Autodesk Fusion 360 part; units mm, degrees
(part 2 of 2)
sketch "Sketch18" plane through (0, 0, 0) normal (0, 0, -1) x (1, 0, 0)
  line L0 (46, -5.5) -> (46, -9.25)
  line L1 (46, -9.25) -> (49.5, -10.5)
  line L2 (49.5, -10.5) -> (65.5, -10.5)
  line L3 (65.5, -10.5) -> (65.5, 45.5)
  line L4 (65.5, 45.5) -> (40.5, 80.5)
  line L5 (40.5, 80.5) -> (-10.5, 80.5)
  line L6 (-10.5, 80.5) -> (-35.5, 45.5)
  line L7 (-35.5, 45.5) -> (-35.5, -10.5)
  line L8 (-35.5, -10.5) -> (-19.5, -10.5)
  line L9 (-19.5, -10.5) -> (-16, -9.25)
  line L10 (-16, -9.25) -> (-16, -5.5)
  line L11 (-16, -5.5) -> (46, -5.5)
  line L12 (35.5, 12.5) -> (33, 24.5)
  line L13 (33, 24.5) -> (49.5, 29.5)
  line L14 (49.5, 29.5) -> (49.5, 5.5)
  line L15 (49.5, 5.5) -> (35.5, 12.5)
  line L16 (27, 75.5) -> (35.5, 75.5)
  line L17 (35.5, 75.5) -> (35.5, 64.5)
  line L18 (35.5, 64.5) -> (27, 64.5)
  line L19 (27, 64.5) -> (27, 75.5)
  line L20 (54.5, 0.5) -> (60.5, 0.5)
  line L21 (60.5, 0.5) -> (60.5, -5.5)
  line L22 (60.5, -5.5) -> (54.5, -5.5)
  line L23 (54.5, -5.5) -> (54.5, 0.5)
  line L24 (54.5, 40.5) -> (60.5, 40.5)
  line L25 (60.5, 40.5) -> (60.5, 34.5)
  line L26 (60.5, 34.5) -> (54.5, 34.5)
  line L27 (54.5, 34.5) -> (54.5, 40.5)
  line L28 (-30.5, 0.5) -> (-24.5, 0.5)
  line L29 (-24.5, 0.5) -> (-24.5, -5.5)
  line L30 (-24.5, -5.5) -> (-30.5, -5.5)
  line L31 (-30.5, -5.5) -> (-30.5, 0.5)
  line L32 (-0.5, 7.5) -> (7.5, 7.5)
  line L33 (7.5, 7.5) -> (7.5, -0.5)
  line L34 (7.5, -0.5) -> (-0.5, -0.5)
  line L35 (-0.5, -0.5) -> (-0.5, 7.5)
  line L36 (2, 35.5) -> (28, 35.5)
  line L37 (28, 35.5) -> (28, 29.5)
  line L38 (28, 29.5) -> (2, 29.5)
  line L39 (2, 29.5) -> (2, 35.5)
  line L40 (-30.5, 40.5) -> (-24.5, 40.5)
  line L41 (-24.5, 40.5) -> (-24.5, 34.5)
  line L42 (-24.5, 34.5) -> (-30.5, 34.5)
  line L43 (-30.5, 34.5) -> (-30.5, 40.5)
  line L44 (22.5, 7.5) -> (30.5, 7.5)
  line L45 (30.5, 7.5) -> (30.5, -0.5)
  line L46 (30.5, -0.5) -> (22.5, -0.5)
  line L47 (22.5, -0.5) -> (22.5, 7.5)
  line L48 (-5.5, 75.5) -> (3, 75.5)
  line L49 (3, 75.5) -> (3, 64.5)
  line L50 (3, 64.5) -> (-5.5, 64.5)
  line L51 (-5.5, 64.5) -> (-5.5, 75.5)
  line L52 (33, 40.5) -> (-3, 40.5)
  line L53 (-3, 40.5) -> (8, 59.5)
  line L54 (8, 59.5) -> (22, 59.5)
  line L55 (22, 59.5) -> (33, 40.5)
  line L56 (-5.5, 12.5) -> (-19.5, 5.5)
  line L57 (-19.5, 5.5) -> (-19.5, 29.5)
  line L58 (-19.5, 29.5) -> (-3, 24.5)
  line L59 (-3, 24.5) -> (-5.5, 12.5)
  line L60 (30.5, -0.5) -> (35.5, -0.5) construction
  line L61 (35.5, -0.5) -> (35.5, -5.5) construction
  line L62 (35.5, -5.5) -> (30.5, -5.5) construction
  line L63 (30.5, -5.5) -> (30.5, -0.5) construction
  line L64 (35.5, -5.5) -> (17.5, -5.5) construction
  line L65 (17.5, -5.5) -> (17.5, 12.5) construction
  line L66 (17.5, 12.5) -> (35.5, 12.5) construction
  line L67 (35.5, 12.5) -> (35.5, -5.5) construction
  line L68 (7.5, -0.5) -> (12.5, -0.5) construction
  line L69 (12.5, -0.5) -> (12.5, -5.5) construction
  line L70 (12.5, -5.5) -> (7.5, -5.5) construction
  line L71 (7.5, -5.5) -> (7.5, -0.5) construction
  line L72 (12.5, -5.5) -> (-5.5, -5.5) construction
  line L73 (-5.5, -5.5) -> (-5.5, 12.5) construction
  line L74 (-5.5, 12.5) -> (12.5, 12.5) construction
  line L75 (12.5, 12.5) -> (12.5, -5.5) construction
  line L76 (-24.5, -5.5) -> (-19.5, -5.5) construction
  line L77 (-19.5, -5.5) -> (-19.5, -10.5) construction
  line L78 (-19.5, -10.5) -> (-24.5, -10.5) construction
  line L79 (-24.5, -10.5) -> (-24.5, -5.5) construction
  line L80 (-19.5, -10.5) -> (-35.5, -10.5) construction
  line L81 (-35.5, -10.5) -> (-35.5, 5.5) construction
  line L82 (-35.5, 5.5) -> (-19.5, 5.5) construction
  line L83 (-19.5, 5.5) -> (-19.5, -10.5) construction
  line L84 (-19.5, 29.5) -> (-35.5, 29.5)
  line L85 (-35.5, 29.5) -> (-35.5, 5.5)
  line L86 (-35.5, 5.5) -> (-19.5, 5.5)
  line L87 (-19.5, 5.5) -> (-19.5, 29.5)
  line L88 (49.5, 29.5) -> (65.5, 29.5)
  line L89 (65.5, 29.5) -> (65.5, 5.5)
  line L90 (65.5, 5.5) -> (49.5, 5.5)
  line L91 (49.5, 5.5) -> (49.5, 29.5)
  line L92 (60.5, 34.5) -> (65.5, 34.5) construction
  line L93 (65.5, 34.5) -> (65.5, 29.5) construction
  line L94 (65.5, 29.5) -> (60.5, 29.5) construction
  line L95 (60.5, 29.5) -> (60.5, 34.5) construction
  line L96 (65.5, 29.5) -> (49, 29.5) construction
  line L97 (49, 29.5) -> (49, 46) construction
  line L98 (49, 46) -> (65.5, 46) construction
  line L99 (65.5, 46) -> (65.5, 29.5) construction
  line L100 (27, 75.5) -> (22, 75.5) construction
  line L101 (22, 75.5) -> (22, 80.5) construction
  line L102 (22, 80.5) -> (27, 80.5) construction
  line L103 (27, 80.5) -> (27, 75.5) construction
  line L104 (22, 80.5) -> (40.5, 80.5) construction
  line L105 (40.5, 80.5) -> (40.5, 59.5) construction
  line L106 (40.5, 59.5) -> (22, 59.5) construction
  line L107 (22, 59.5) -> (22, 80.5) construction
  line L108 (49, 29.5) -> (31.25, 59.5)
  line L109 (40.5, 80.5) -> (40.5, 59.5)
  line L110 (40.5, 59.5) -> (31.25, 59.5)
  line L111 (-5.5, 75.5) -> (-10.5, 75.5) construction
  line L112 (-10.5, 75.5) -> (-10.5, 80.5) construction
  line L113 (-10.5, 80.5) -> (-5.5, 80.5) construction
  line L114 (-5.5, 80.5) -> (-5.5, 75.5) construction
  line L115 (-10.5, 80.5) -> (8, 80.5) construction
  line L116 (8, 80.5) -> (8, 59.5) construction
  line L117 (8, 59.5) -> (-10.5, 59.5) construction
  line L118 (-10.5, 59.5) -> (-10.5, 80.5) construction
  line L119 (22, 59.5) -> (8, 59.5)
  line L120 (8, 59.5) -> (8, 80.5)
  line L121 (8, 80.5) -> (22, 80.5)
  line L122 (22, 80.5) -> (22, 59.5)
  line L123 (-35.5, 29.5) -> (-19.5, 29.5) construction
  line L124 (-19.5, 29.5) -> (-19.5, 45.5) construction
  line L125 (-19.5, 45.5) -> (-35.5, 45.5) construction
  line L126 (-35.5, 45.5) -> (-35.5, 29.5) construction
  line L127 (-19.5, 29.5) -> (-1.25, 59.5)
  line L128 (49, 29.5) -> (49, 46)
  line L129 (49, 46) -> (65.5, 46)
  line L130 (-1.25, 59.5) -> (-10.5, 59.5)
  line L131 (-10.5, 59.5) -> (-10.5, 80.5)
  line L132 (-19.5, 29.5) -> (-19.5, 45.5)
  line L133 (-19.5, 45.5) -> (-35.5, 45.5)
  line L134 (49, 46) -> (-19.5, 45.5)
  line L135 (49, 46) -> (-19.5, 45.5)
  dimension "d166" = 5
  dimension "d167" = 5
  dimension "d168" = 18
  dimension "d169" = 18
  dimension "d170" = 5
  dimension "d171" = 18
  dimension "d172" = 18
  dimension "d173" = 16
  dimension "d174" = 16
  dimension "d175" = 16.5
  dimension "d176" = 16.5
  dimension "d177" = 5
  dimension "d178" = 18.5
  dimension "d179" = 21
  dimension "d180" = 18.5
  dimension "d181" = 21
  dimension "d182" = 16
  dimension "d183" = 16
  constraint horizontal L60
  constraint vertical L61
  constraint horizontal L62
  constraint vertical L63
  constraint coincident L45.end L46.start
  constraint horizontal L64
  constraint vertical L65
  constraint horizontal L66
  constraint vertical L67
  constraint horizontal L68
  constraint vertical L69
  constraint horizontal L70
  constraint vertical L71
  constraint coincident L33.end L34.start
  constraint horizontal L72
  constraint vertical L73
  constraint horizontal L74
  constraint vertical L75
  constraint horizontal L76
  constraint vertical L77
  constraint horizontal L78
  constraint vertical L79
  constraint coincident L8.end L9.start
  constraint coincident L29.end L30.start
  constraint horizontal L80
  constraint vertical L81
  constraint horizontal L82
  constraint vertical L83
  constraint horizontal L84
  constraint vertical L85
  constraint horizontal L86
  constraint vertical L87
  constraint coincident L57.end L58.start
  constraint horizontal L88
  constraint vertical L89
  constraint horizontal L90
  constraint vertical L91
  constraint coincident L3 L89.end
  constraint coincident L13.end L14.start
  constraint horizontal L92
  constraint vertical L93
  constraint horizontal L94
  constraint vertical L95
  constraint coincident L25.end L26.start
  constraint horizontal L96
  constraint vertical L97
  constraint horizontal L98
  constraint vertical L99
  constraint horizontal L100
  constraint vertical L101
  constraint horizontal L102
  constraint vertical L103
  constraint coincident L16.start L19.end
  constraint horizontal L104
  constraint vertical L105
  constraint horizontal L106
  constraint vertical L107
  constraint midpoint L106 L108.end
  constraint horizontal L111
  constraint vertical L112
  constraint horizontal L113
  constraint vertical L114
  constraint coincident L5.end L6.start
  constraint coincident L48.start L51.end
  constraint horizontal L115
  constraint vertical L116
  constraint horizontal L117
  constraint vertical L118
  constraint horizontal L119
  constraint vertical L120
  constraint horizontal L121
  constraint vertical L122
  constraint coincident L54.end L55.start
  constraint horizontal L123
  constraint vertical L124
  constraint horizontal L125
  constraint vertical L126
  constraint midpoint L117 L127.end
  constraint coincident L6.end L7.start
  measures "d166" distance of L45.end L60.end
  measures "d167" distance of L45.end L62.end
  measures "d168" distance of L61.end L64.end
  measures "d169" distance of L61.end L12.start
  measures "d170" distance of L33.end L68.end
  measures "d171" distance of L69.end L72.end
  measures "d172" distance of L69.end L74.end
  measures "d173" distance of L8.end L7.end
  measures "d174" distance of L8.end L56.end
  measures "d175" distance of L88.end L96.end
  measures "d176" distance of L88.end L98.end
  measures "d177" distance of L16.start L100.end
  measures "d178" distance of L101.end L4.end
  measures "d179" distance of L101.end L54.end
  measures "d180" distance of L5.end L115.end
  measures "d181" distance of L5.end L117.end
  measures "d182" distance of L84.end L57.end
  measures "d183" distance of L84.end L6.end
extrude "Extrude22" cut sketch "Sketch18" against normal blind 6 contours L3 L14 L88 L89 L90 L91 | L7 L57 L84 L85 L86 L87 | L4 L108 L109 L110 L129 L134 L135 | L6 L127 L130 L131 L133 L134 L135 | L5 L54 L119 L120 L121 L122
sketch "Sketch19" plane through (0, 0, 0) normal (0, 0, -1) x (1, 0, 0)
  line L0 (40.5, 59.5) -> (40.5, 80.5)
  line L1 (40.5, 80.5) -> (22, 80.5)
  line L2 (22, 80.5) -> (22, 59.5)
  line L3 (22, 59.5) -> (33, 40.5)
  line L4 (33, 40.5) -> (-3, 40.5)
  line L5 (-3, 40.5) -> (8, 59.5)
  line L6 (8, 59.5) -> (8, 80.5)
  line L7 (8, 80.5) -> (-10.5, 80.5)
  line L8 (-10.5, 80.5) -> (-10.5, 59.5)
  line L9 (-10.5, 59.5) -> (-1.25, 59.5)
  line L10 (-1.25, 59.5) -> (-9.7233, 45.5714)
  line L11 (-9.7233, 45.5714) -> (-19.5, 45.5)
  line L12 (-19.5, 45.5) -> (-35.5, 45.5)
  line L13 (-35.5, 45.5) -> (-35.5, 29.5)
  line L14 (-35.5, 29.5) -> (-19.5, 29.5)
  line L15 (-19.5, 29.5) -> (-3, 24.5)
  line L16 (-3, 24.5) -> (-5.5, 12.5)
  line L17 (-5.5, 12.5) -> (-19.5, 5.5)
  line L18 (-19.5, 5.5) -> (-35.5, 5.5)
  line L19 (-35.5, 5.5) -> (-35.5, -10.5)
  line L20 (-35.5, -10.5) -> (-19.5, -10.5)
  line L21 (-19.5, -10.5) -> (-16, -9.25)
  line L22 (-16, -9.25) -> (-16, -5.5)
  line L23 (-16, -5.5) -> (46, -5.5)
  line L24 (46, -5.5) -> (46, -9.25)
  line L25 (46, -9.25) -> (49.5, -10.5)
  line L26 (49.5, -10.5) -> (65.5, -10.5)
  line L27 (65.5, -10.5) -> (65.5, 5.5)
  line L28 (65.5, 5.5) -> (49.5, 5.5)
  line L29 (49.5, 5.5) -> (35.5, 12.5)
  line L30 (35.5, 12.5) -> (33, 24.5)
  line L31 (33, 24.5) -> (49.5, 29.5)
  line L32 (49.5, 29.5) -> (65.5, 29.5)
  line L33 (65.5, 29.5) -> (65.5, 45.5)
  line L34 (65.5, 45.5) -> (65.1429, 46)
  line L35 (65.1429, 46) -> (49, 46)
  line L36 (49, 46) -> (39.2795, 45.929)
  line L37 (39.2795, 45.929) -> (31.25, 59.5)
  line L38 (31.25, 59.5) -> (40.5, 59.5)
  line L39 (27, 75.5) -> (35.5, 75.5)
  line L40 (35.5, 75.5) -> (35.5, 64.5)
  line L41 (35.5, 64.5) -> (27, 64.5)
  line L42 (27, 64.5) -> (27, 75.5)
  line L43 (54.5, 0.5) -> (60.5, 0.5)
  line L44 (60.5, 0.5) -> (60.5, -5.5)
  line L45 (60.5, -5.5) -> (54.5, -5.5)
  line L46 (54.5, -5.5) -> (54.5, 0.5)
  line L47 (54.5, 40.5) -> (60.5, 40.5)
  line L48 (60.5, 40.5) -> (60.5, 34.5)
  line L49 (60.5, 34.5) -> (54.5, 34.5)
  line L50 (54.5, 34.5) -> (54.5, 40.5)
  line L51 (-30.5, 0.5) -> (-24.5, 0.5)
  line L52 (-24.5, 0.5) -> (-24.5, -5.5)
  line L53 (-24.5, -5.5) -> (-30.5, -5.5)
  line L54 (-30.5, -5.5) -> (-30.5, 0.5)
  line L55 (-0.5, 7.5) -> (7.5, 7.5)
  line L56 (7.5, 7.5) -> (7.5, -0.5)
  line L57 (7.5, -0.5) -> (-0.5, -0.5)
  line L58 (-0.5, -0.5) -> (-0.5, 7.5)
  line L59 (2, 35.5) -> (28, 35.5)
  line L60 (28, 35.5) -> (28, 29.5)
  line L61 (28, 29.5) -> (2, 29.5)
  line L62 (2, 29.5) -> (2, 35.5)
  line L63 (-30.5, 40.5) -> (-24.5, 40.5)
  line L64 (-24.5, 40.5) -> (-24.5, 34.5)
  line L65 (-24.5, 34.5) -> (-30.5, 34.5)
  line L66 (-30.5, 34.5) -> (-30.5, 40.5)
  line L67 (22.5, 7.5) -> (30.5, 7.5)
  line L68 (30.5, 7.5) -> (30.5, -0.5)
  line L69 (30.5, -0.5) -> (22.5, -0.5)
  line L70 (22.5, -0.5) -> (22.5, 7.5)
  line L71 (-5.5, 75.5) -> (3, 75.5)
  line L72 (3, 75.5) -> (3, 64.5)
  line L73 (3, 64.5) -> (-5.5, 64.5)
  line L74 (-5.5, 64.5) -> (-5.5, 75.5)
  line L75 (7.5, 7.5) -> (12.5, 7.5) construction
  line L76 (12.5, 7.5) -> (12.5, 12.5) construction
  line L77 (12.5, 12.5) -> (7.5, 12.5) construction
  line L78 (7.5, 12.5) -> (7.5, 7.5) construction
  line L79 (12.5, 12.5) -> (-5.5, 12.5) construction
  line L80 (-5.5, 12.5) -> (-5.5, -5.5) construction
  line L81 (-5.5, -5.5) -> (12.5, -5.5) construction
  line L82 (12.5, -5.5) -> (12.5, 12.5) construction
  line L83 (30.5, -0.5) -> (35.5, -0.5) construction
  line L84 (35.5, -0.5) -> (35.5, -5.5) construction
  line L85 (35.5, -5.5) -> (30.5, -5.5) construction
  line L86 (30.5, -5.5) -> (30.5, -0.5) construction
  line L87 (35.5, -5.5) -> (17.5, -5.5) construction
  line L88 (17.5, -5.5) -> (17.5, 12.5) construction
  line L89 (17.5, 12.5) -> (35.5, 12.5) construction
  line L90 (35.5, 12.5) -> (35.5, -5.5) construction
  line L91 (2, 35.5) -> (-3, 35.5) construction
  line L92 (-3, 35.5) -> (-3, 40.5) construction
  line L93 (-3, 40.5) -> (2, 40.5) construction
  line L94 (2, 40.5) -> (2, 35.5) construction
  line L95 (-3, 40.5) -> (33, 40.5) construction
  line L96 (33, 40.5) -> (33, 24.5) construction
  line L97 (33, 24.5) -> (-3, 24.5) construction
  line L98 (-3, 24.5) -> (-3, 40.5) construction
  line L99 (-3, 24.5) -> (2, 24.5) construction
  line L100 (33, 24.5) -> (28, 24.5) construction
  line L101 (2, 24.5) -> (12.5, 12.5)
  line L102 (17.5, 12.5) -> (12.5, 12.5)
  line L103 (17.5, 12.5) -> (28, 24.5)
  line L104 (28, 24.5) -> (2, 24.5)
  dimension "d186" = 5
  dimension "d187" = 5
  dimension "d188" = 18
  dimension "d189" = 5
  dimension "d190" = 18
  dimension "d191" = 18
  dimension "d192" = 36
  dimension "d193" = 16
  dimension "d194" = 5
  dimension "d195" = 5
  constraint horizontal L75
  constraint vertical L76
  constraint horizontal L77
  constraint vertical L78
  constraint coincident L55.end L56.start
  constraint horizontal L79
  constraint vertical L80
  constraint horizontal L81
  constraint vertical L82
  constraint horizontal L83
  constraint vertical L84
  constraint horizontal L85
  constraint vertical L86
  constraint coincident L68.end L69.start
  constraint horizontal L87
  constraint vertical L88
  constraint horizontal L89
  constraint vertical L90
  constraint horizontal L91
  constraint vertical L92
  constraint horizontal L93
  constraint vertical L94
  constraint coincident L4.end L5.start
  constraint coincident L59.start L62.end
  constraint horizontal L95
  constraint vertical L96
  constraint horizontal L97
  constraint vertical L98
  constraint perpendicular L98 L99
  constraint perpendicular L96 L100
  measures "d186" distance of L55.end L75.end
  measures "d187" distance of L55.end L77.end
  measures "d188" distance of L76.end L16.end
  measures "d189" distance of L68.end L83.end
  measures "d190" distance of L84.end L87.end
  measures "d191" distance of L84.end L29.end
  measures "d192" distance of L4.end L3.end
  measures "d193" distance of L4.end L15.end
  measures "d194" distance of L15.end L99.end
  measures "d195" distance of L30.end L100.end
extrude "Extrude23" cut sketch "Sketch19" against normal blind 6 contours L101 L102 L103 L104
sketch "Sketch20" plane through (0, 0, 0) normal (0, 0, -1) x (1, 0, 0)
  line L0 (2, 24.5) -> (28, 24.5)
  line L1 (28, 24.5) -> (17.5, 12.5)
  line L2 (17.5, 12.5) -> (12.5, 12.5)
  line L3 (12.5, 12.5) -> (2, 24.5)
  line L4 (40.5, 59.5) -> (40.5, 80.5)
  line L5 (40.5, 80.5) -> (22, 80.5)
  line L6 (22, 80.5) -> (22, 59.5)
  line L7 (22, 59.5) -> (33, 40.5)
  line L8 (33, 40.5) -> (-3, 40.5)
  line L9 (-3, 40.5) -> (8, 59.5)
  line L10 (8, 59.5) -> (8, 80.5)
  line L11 (8, 80.5) -> (-10.5, 80.5)
  line L12 (-10.5, 80.5) -> (-10.5, 59.5)
  line L13 (-10.5, 59.5) -> (-1.25, 59.5)
  line L14 (-1.25, 59.5) -> (-9.7233, 45.5714)
  line L15 (-9.7233, 45.5714) -> (-19.5, 45.5)
  line L16 (-19.5, 45.5) -> (-35.5, 45.5)
  line L17 (-35.5, 45.5) -> (-35.5, 29.5)
  line L18 (-35.5, 29.5) -> (-19.5, 29.5)
  line L19 (-19.5, 29.5) -> (-3, 24.5)
  line L20 (-3, 24.5) -> (-5.5, 12.5)
  line L21 (-5.5, 12.5) -> (-19.5, 5.5)
  line L22 (-19.5, 5.5) -> (-35.5, 5.5)
  line L23 (-35.5, 5.5) -> (-35.5, -10.5)
  line L24 (-35.5, -10.5) -> (-19.5, -10.5)
  line L25 (-19.5, -10.5) -> (-16, -9.25)
  line L26 (-16, -9.25) -> (-16, -5.5)
  line L27 (-16, -5.5) -> (46, -5.5)
  line L28 (46, -5.5) -> (46, -9.25)
  line L29 (46, -9.25) -> (49.5, -10.5)
  line L30 (49.5, -10.5) -> (65.5, -10.5)
  line L31 (65.5, -10.5) -> (65.5, 5.5)
  line L32 (65.5, 5.5) -> (49.5, 5.5)
  line L33 (49.5, 5.5) -> (35.5, 12.5)
  line L34 (35.5, 12.5) -> (33, 24.5)
  line L35 (33, 24.5) -> (49.5, 29.5)
  line L36 (49.5, 29.5) -> (65.5, 29.5)
  line L37 (65.5, 29.5) -> (65.5, 45.5)
  line L38 (65.5, 45.5) -> (65.1429, 46)
  line L39 (65.1429, 46) -> (49, 46)
  line L40 (49, 46) -> (39.2795, 45.929)
  line L41 (39.2795, 45.929) -> (31.25, 59.5)
  line L42 (31.25, 59.5) -> (40.5, 59.5)
  line L43 (27, 75.5) -> (35.5, 75.5)
  line L44 (35.5, 75.5) -> (35.5, 64.5)
  line L45 (35.5, 64.5) -> (27, 64.5)
  line L46 (27, 64.5) -> (27, 75.5)
  line L47 (54.5, 0.5) -> (60.5, 0.5)
  line L48 (60.5, 0.5) -> (60.5, -5.5)
  line L49 (60.5, -5.5) -> (54.5, -5.5)
  line L50 (54.5, -5.5) -> (54.5, 0.5)
  line L51 (54.5, 40.5) -> (60.5, 40.5)
  line L52 (60.5, 40.5) -> (60.5, 34.5)
  line L53 (60.5, 34.5) -> (54.5, 34.5)
  line L54 (54.5, 34.5) -> (54.5, 40.5)
  line L55 (-30.5, 0.5) -> (-24.5, 0.5)
  line L56 (-24.5, 0.5) -> (-24.5, -5.5)
  line L57 (-24.5, -5.5) -> (-30.5, -5.5)
  line L58 (-30.5, -5.5) -> (-30.5, 0.5)
  line L59 (-0.5, 7.5) -> (7.5, 7.5)
  line L60 (7.5, 7.5) -> (7.5, -0.5)
  line L61 (7.5, -0.5) -> (-0.5, -0.5)
  line L62 (-0.5, -0.5) -> (-0.5, 7.5)
  line L63 (2, 35.5) -> (28, 35.5)
  line L64 (28, 35.5) -> (28, 29.5)
  line L65 (28, 29.5) -> (2, 29.5)
  line L66 (2, 29.5) -> (2, 35.5)
  line L67 (-30.5, 40.5) -> (-24.5, 40.5)
  line L68 (-24.5, 40.5) -> (-24.5, 34.5)
  line L69 (-24.5, 34.5) -> (-30.5, 34.5)
  line L70 (-30.5, 34.5) -> (-30.5, 40.5)
  line L71 (22.5, 7.5) -> (30.5, 7.5)
  line L72 (30.5, 7.5) -> (30.5, -0.5)
  line L73 (30.5, -0.5) -> (22.5, -0.5)
  line L74 (22.5, -0.5) -> (22.5, 7.5)
  line L75 (-5.5, 75.5) -> (3, 75.5)
  line L76 (3, 75.5) -> (3, 64.5)
  line L77 (3, 64.5) -> (-5.5, 64.5)
  line L78 (-5.5, 64.5) -> (-5.5, 75.5)
  line L79 (65.5, 29.5) -> (49, 29.5) construction
  line L80 (49, 29.5) -> (49, 46) construction
  line L81 (49, 46) -> (65.5, 46) construction
  line L82 (65.5, 46) -> (65.5, 29.5) construction
  line L83 (49, 29.5) -> (49, 34.5)
  line L84 (49, 46) -> (49, 41)
  line L85 (28, 29.5) -> (33, 29.5) construction
  line L86 (33, 29.5) -> (33, 35.5) construction
  line L87 (33, 35.5) -> (28, 35.5) construction
  line L88 (28, 35.5) -> (28, 29.5) construction
  line L89 (49, 34.5) -> (33, 29.5)
  line L90 (49, 41) -> (49, 34.5)
  line L91 (49, 41) -> (33, 35.5)
  line L92 (33, 35.5) -> (33, 29.5)
  line L93 (2, 29.5) -> (-3, 29.5) construction
  line L94 (-3, 29.5) -> (-3, 35.5) construction
  line L95 (-3, 35.5) -> (2, 35.5) construction
  line L96 (2, 35.5) -> (2, 29.5) construction
  line L97 (-19.5, 29.5) -> (-19.5, 45.5) construction
  line L98 (-19.5, 45.5) -> (-19.4635, 40.5001) construction
  line L99 (-19.4635, 40.5001) -> (-19.4635, 34.5001) construction
  line L100 (-19.4635, 40.5001) -> (-3, 35.5)
  line L101 (-3, 35.5) -> (-3, 29.5)
  line L102 (-3, 29.5) -> (-19.4635, 34.5001)
  line L103 (-19.4635, 34.5001) -> (-19.4635, 40.5001)
  line L104 (-35.5, -10.5) -> (-19.5, -10.5) construction
  line L105 (-19.5, -10.5) -> (-19.5, 5.5) construction
  line L106 (-19.5, 5.5) -> (-35.5, 5.5) construction
  line L107 (-35.5, 5.5) -> (-35.5, -10.5) construction
  line L108 (65.5, -10.5) -> (49.5, -10.5) construction
  line L109 (49.5, -10.5) -> (49.5, 5.5) construction
  line L110 (49.5, 5.5) -> (65.5, 5.5) construction
  line L111 (65.5, 5.5) -> (65.5, -10.5) construction
  line L112 (30.5, -0.5) -> (35.5, -0.5) construction
  line L113 (35.5, -0.5) -> (35.5, -5.5) construction
  line L114 (35.5, -5.5) -> (30.5, -5.5) construction
  line L115 (30.5, -5.5) -> (30.5, -0.5) construction
  line L116 (35.5, -5.5) -> (17.5, -5.5) construction
  line L117 (17.5, -5.5) -> (17.5, 12.5) construction
  line L118 (17.5, 12.5) -> (35.5, 12.5) construction
  line L119 (35.5, 12.5) -> (35.5, -5.5) construction
  line L120 (12.5, 12.5) -> (-5.5, 12.5) construction
  line L121 (-5.5, 12.5) -> (-5.5, -5.5) construction
  line L122 (-5.5, -5.5) -> (12.5, -5.5) construction
  line L123 (12.5, -5.5) -> (12.5, 12.5) construction
  line L124 (-0.5, -0.5) -> (-5.5, -0.5) construction
  line L125 (-5.5, -0.5) -> (-5.5, 7.5) construction
  line L126 (-5.5, 7.5) -> (-0.5, 7.5) construction
  line L127 (-0.5, 7.5) -> (-0.5, -0.5) construction
  line L128 (30.5, -0.5) -> (35.5, -0.5) construction
  line L129 (35.5, -0.5) -> (35.5, 7.5) construction
  line L130 (35.5, 7.5) -> (30.5, 7.5) construction
  line L131 (30.5, 7.5) -> (30.5, -0.5) construction
  line L132 (35.5, 7.5) -> (49.5, -2.5)
  line L133 (49.5, -2.5) -> (35.5, -0.5)
  line L134 (35.5, 7.5) -> (35.5, -0.5)
  line L135 (-5.5, -0.5) -> (-5.5, 7.5)
  line L136 (-5.5, 7.5) -> (-19.5, -2.5)
  line L137 (-5.5, -0.5) -> (-19.5, -2.5)
  line L138 (17.5, 12.5) -> (12.5, 12.5)
  line L139 (12.5, 12.5) -> (12.5, -5.5)
  line L140 (12.5, -5.5) -> (17.5, -5.5)
  line L141 (17.5, -5.5) -> (17.5, 12.5)
  dimension "d198" = 5
  dimension "d199" = 5
  dimension "d200" = 5
  dimension "d201" = 6
  dimension "d202" = 5
  dimension "d203" = 6
  dimension "d204" = 5
  dimension "d205" = 6
  dimension "d206" = 5
  dimension "d207" = 18
  dimension "d208" = 18
  dimension "d209" = 18
  dimension "d210" = 8
  dimension "d211" = 8
  constraint horizontal L79
  constraint vertical L80
  constraint horizontal L81
  constraint vertical L82
  constraint coincident L39.end L40.start
  constraint coincident L36.end L37.start
  constraint perpendicular L36 L83
  constraint perpendicular L39 L84
  constraint horizontal L85
  constraint vertical L86
  constraint horizontal L87
  constraint vertical L88
  constraint coincident L64.end L65.start
  constraint horizontal L93
  constraint vertical L94
  constraint horizontal L95
  constraint vertical L96
  constraint coincident L65.end L66.start
  constraint coincident L18.end L19.start
  constraint coincident L15.end L16.start
  constraint perpendicular L15 L98
  constraint perpendicular L18 L99
  constraint horizontal L104
  constraint vertical L105
  constraint horizontal L106
  constraint vertical L107
  constraint coincident L21.end L22.start
  constraint coincident L23.end L24.start
  constraint horizontal L108
  constraint vertical L109
  constraint horizontal L110
  constraint vertical L111
  constraint coincident L32.end L33.start
  constraint coincident L30.end L31.start
  constraint horizontal L112
  constraint vertical L113
  constraint horizontal L114
  constraint vertical L115
  constraint coincident L72.end L73.start
  constraint horizontal L116
  constraint vertical L117
  constraint horizontal L118
  constraint vertical L119
  constraint horizontal L120
  constraint vertical L121
  constraint horizontal L122
  constraint vertical L123
  constraint coincident L2.end L3.start
  constraint horizontal L124
  constraint vertical L125
  constraint horizontal L126
  constraint vertical L127
  constraint coincident L61.end L62.start
  constraint horizontal L128
  constraint vertical L129
  constraint horizontal L130
  constraint vertical L131
  constraint midpoint L109 L132.end
  constraint midpoint L105 L136.end
  constraint horizontal L138
  constraint vertical L139
  constraint horizontal L140
  constraint vertical L141
  measures "d198" distance of L79.end L83.end
  measures "d199" distance of L39.end L84.end
  measures "d200" distance of L64.end L85.end
  measures "d201" distance of L64.end L63.end
  measures "d202" distance of L65.end L93.end
  measures "d203" distance of L65.end L63.start
  measures "d204" distance of L15.end L98.end
  measures "d205" distance of L98.end L99.end
  measures "d206" distance of L72.end L112.end
  measures "d207" distance of L113.end L116.end
  measures "d208" distance of L113.end L33.end
  measures "d209" distance of L2.end L20.end
  measures "d210" distance of L61.end L59.start
  measures "d211" distance of L72.end L71.end
extrude "Extrude24" cut sketch "Sketch20" against normal blind 6 contours L2 L27 L138 L139 L140 L141 | L89 L90 L91 L92 | L100 L101 L102 L103 | L132 L133 L134 | L135 L136 L137
sketch "Sketch21" plane through (-16, 0, 0) normal (-1, 0, 0) x (0, -1, 0)
  line L0 (11.5, 6) -> (11.5, 36)
  line L1 (11.5, 36) -> (-18.5, 36)
  line L2 (-18.5, 36) -> (-18.5, -9)
  line L3 (-18.5, -9) -> (-5.5, -9)
  line L4 (-5.5, -9) -> (-5.5, 0)
  line L5 (-5.5, 0) -> (-9.25, 0)
  line L6 (-9.25, 0) -> (-9.25, 6)
  line L7 (-9.25, 6) -> (-2, 6)
  line L8 (-2, 6) -> (0, 6)
  line L9 (0, 6) -> (7.25, 6)
  line L10 (7.25, 6) -> (11.5, 6)
  line L11 (-18.5, 36) -> (-13.5, 36) construction
  line L12 (-13.5, 36) -> (-13.5, 31) construction
  line L13 (-13.5, 31) -> (-18.5, 31) construction
  line L14 (-18.5, 31) -> (-18.5, 36) construction
  line L15 (11.5, 6) -> (6.5, 6) construction
  line L16 (6.5, 6) -> (6.5, 11) construction
  line L17 (6.5, 11) -> (11.5, 11) construction
  line L18 (11.5, 11) -> (11.5, 6) construction
  line L19 (6.5, 11) -> (2.5, 11) construction
  line L20 (2.5, 11) -> (2.5, 15) construction
  line L21 (2.5, 15) -> (6.5, 15) construction
  line L22 (6.5, 15) -> (6.5, 11) construction
  line L23 (-13.5, 31) -> (-9.5, 31) construction
  line L24 (-9.5, 31) -> (-9.5, 27) construction
  line L25 (-9.5, 27) -> (-13.5, 27) construction
  line L26 (-13.5, 27) -> (-13.5, 31) construction
  line L27 (-13.5, 27) -> (-13.5, 31)
  line L28 (-13.5, 27) -> (2.5, 11)
  line L29 (6.5, 15) -> (-9.5, 31)
  line L30 (-13.5, 31) -> (6.5, 31)
  line L31 (6.5, 31) -> (6.5, 11)
  line L32 (6.5, 11) -> (-13.5, 11)
  line L33 (-13.5, 11) -> (-13.5, 27)
  dimension "d214" = 5
  dimension "d215" = 5
  dimension "d216" = 5
  dimension "d217" = 5
  dimension "d218" = 4
  dimension "d219" = 4
  dimension "d220" = 4
  dimension "d221" = 20
  constraint horizontal L11
  constraint vertical L12
  constraint horizontal L13
  constraint vertical L14
  constraint coincident L1.end L2.start
  constraint horizontal L15
  constraint vertical L16
  constraint horizontal L17
  constraint vertical L18
  constraint coincident L0.start L10.end
  constraint horizontal L19
  constraint vertical L20
  constraint horizontal L21
  constraint vertical L22
  constraint horizontal L23
  constraint vertical L24
  constraint horizontal L25
  constraint vertical L26
  constraint perpendicular L24 L30
  constraint perpendicular L19 L31
  constraint perpendicular L31 L32
  measures "d214" distance of L1.end L11.end
  measures "d215" distance of L1.end L13.end
  measures "d216" distance of L0.start L15.end
  measures "d217" distance of L0.start L17.end
  measures "d218" distance of L16.end L19.end
  measures "d219" distance of L12.end L23.end
  measures "d220" distance of L12.end L25.end
  measures "d221" distance of L16.end L32.end
extrude "Extrude25" cut sketch "Sketch21" against normal blind 5 contours L28 L32 L33 | L29 L30 L31
extrude "Extrude26" cut sketch "Sketch21" along normal blind 5 from surface at -62 contours L28 L32 L33 | L29 L30 L31
sketch "Sketch22" plane through (0, 0, 36) normal (0, 0, 1) x (-1, 0, 0)
  line L0 (-46, -18.5) -> (16, -18.5)
  line L1 (16, -18.5) -> (16, 11.5)
  line L2 (16, 11.5) -> (-46, 11.5)
  line L3 (-46, 11.5) -> (-46, -18.5)
  line L4 (-26.75, 10.5) -> (-3.25, 10.5)
  line L5 (-3.25, 10.5) -> (-3.25, -16.5)
  line L6 (-3.25, -16.5) -> (-26.75, -16.5)
  line L7 (-26.75, -16.5) -> (-26.75, 10.5)
  line L8 (16, -18.5) -> (11, -18.5) construction
  line L9 (11, -18.5) -> (11, -13.5) construction
  line L10 (11, -13.5) -> (16, -13.5) construction
  line L11 (16, -13.5) -> (16, -18.5) construction
  line L12 (16, 11.5) -> (11, 11.5) construction
  line L13 (11, 11.5) -> (11, 6.5) construction
  line L14 (11, 6.5) -> (16, 6.5) construction
  line L15 (16, 6.5) -> (16, 11.5) construction
  line L16 (11, 6.5) -> (16, 6.5) construction
  line L17 (16, 6.5) -> (16, -13.5) construction
  line L18 (16, -13.5) -> (11, -13.5) construction
  line L19 (11, -13.5) -> (11, 6.5) construction
  line L20 (11, -13.5) -> (-3.25, -13.5)
  line L21 (-3.25, -13.5) -> (-3.25, 6.5)
  line L22 (-3.25, 6.5) -> (11, 6.5)
  line L23 (11, 6.5) -> (11, -13.5)
  line L24 (-3.25, -13.5) -> (-26.75, -13.5) construction
  line L25 (-26.75, -13.5) -> (-41, -13.5)
  line L26 (-41, -13.5) -> (-41, 6.5)
  line L27 (-41, 6.5) -> (-26.75, 6.5)
  line L28 (-26.75, 6.5) -> (-26.75, -13.5)
  dimension "d227" = 5
  dimension "d228" = 5
  dimension "d229" = 5
  dimension "d230" = 5
  dimension "d231" = 14.25
  dimension "d232" = 20
  dimension "d233" = 14.25
  dimension "d234" = 20
  constraint horizontal L8
  constraint vertical L9
  constraint horizontal L10
  constraint vertical L11
  constraint coincident L0.end L1.start
  constraint horizontal L12
  constraint vertical L13
  constraint horizontal L14
  constraint vertical L15
  constraint coincident L1.end L2.start
  constraint horizontal L16
  constraint vertical L17
  constraint horizontal L18
  constraint vertical L19
  constraint horizontal L20
  constraint vertical L21
  constraint horizontal L22
  constraint vertical L23
  constraint coincident L7 L24.end
  constraint perpendicular L7 L24
  constraint horizontal L25
  constraint vertical L26
  constraint horizontal L27
  constraint vertical L28
  measures "d227" distance of L0.end L8.end
  measures "d228" distance of L0.end L10.end
  measures "d229" distance of L1.end L12.end
  measures "d230" distance of L1.end L14.end
  measures "d231" distance of L9.end L20.end
  measures "d232" distance of L9.end L13.end
  measures "d233" distance of L24.end L25.end
  measures "d234" distance of L24.end L27.end
extrude "Extrude27" cut sketch "Sketch22" against normal blind 5 contours L7 L25 L26 L27 L28 | L5 L20 L21 L22 L23
extrude "Extrude28" cut 2 faces at (37.3333, 5.1667, 31) (-7.3333, 5.1667, 31) along direction (0, 0, -1) blind 7
extrude "Extrude29" add 1 faces at (10, 14.5, 21.6667) along direction (0, -1, 0) blind 1
sketch "Sketch23" plane through (0, 13.5, 0) normal (0, -1, 0) x (1, 0, 0)
  line L0 (41, 36) -> (26.75, 36)
  line L1 (26.75, 36) -> (26.75, 31)
  line L2 (26.75, 31) -> (3.25, 31)
  line L3 (3.25, 31) -> (3.25, 36)
  line L4 (3.25, 36) -> (-11, 36)
  line L5 (-11, 36) -> (-11, 27)
  line L6 (-11, 27) -> (-16, 27)
  line L7 (-16, 27) -> (-16, 11)
  line L8 (-16, 11) -> (-11, 11)
  line L9 (-11, 11) -> (-11, 24)
  line L10 (-11, 24) -> (0, 24)
  line L11 (0, 24) -> (0, 17)
  line L12 (0, 17) -> (30, 17)
  line L13 (30, 17) -> (30, 24)
  line L14 (30, 24) -> (41, 24)
  line L15 (41, 24) -> (41, 11)
  line L16 (41, 11) -> (46, 11)
  line L17 (46, 11) -> (46, 27)
  line L18 (46, 27) -> (41, 27)
  line L19 (41, 27) -> (41, 36)
  line L20 (0, 24) -> (-2, 24)
  line L21 (0, 24) -> (0, 22)
  line L22 (4, 31) -> (7, 31)
  line L23 (7, 31) -> (0, 22)
  line L24 (-2, 24) -> (4, 31)
  line L25 (30, 24) -> (30, 22)
  line L26 (30, 24) -> (32, 24)
  line L27 (26, 31) -> (23, 31)
  line L28 (23, 31) -> (30, 22)
  line L29 (26, 31) -> (32, 24)
  dimension "d241" = 2
  dimension "d242" = 2
  dimension "d243" = 3
  constraint coincident L10.end L11.start
  constraint coincident L10 L20.end
  constraint coincident L11 L21.end
  constraint coincident L2 L22.start
  constraint coincident L2 L22.end
  constraint coincident L13.end L14.start
  constraint coincident L13 L25.end
  constraint perpendicular L13 L26
  constraint coincident L2 L27.start
  constraint perpendicular L1 L27
  measures "d241" distance of L13.end L25.end
  measures "d242" distance of L13.end L26.end
  measures "d243" distance of L27.start L27.end
extrude "Extrude30" add sketch "Sketch23" along normal blind 13 contours L2 L13 L14 L25 L26 L27 L28 L29 | L2 L10 L11 L20 L21 L22 L23 L24
